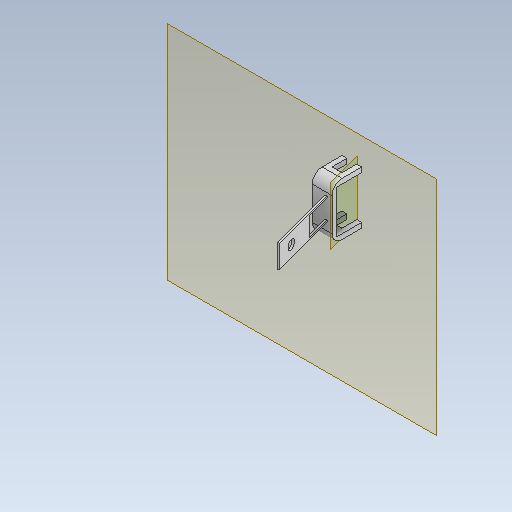
# Autodesk Inventor part: Кранштейн сервомоторов
Saved by Autodesk Inventor 2021.2 (Build 252289000, 289)
## iProperties
Created: 2021-10-14
Part Number: Кранштейн сервомоторов
Material: Типовые
Document SubType Name: Modeling
Designer: Surflay
Density: 1 g/cm^3
Appearance: По умолчанию
Author: Surflay
Autodesk Inventor part; units mm, degrees
ref_plane "YZ Plane" through (0, 0, 0) normal (1, 0, 0) x (0, 1, 0)
ref_plane "XZ Plane" through (0, 0, 0) normal (0, 1, 0) x (-1, 0, 0)
ref_plane "XY Plane" through (0, 0, 0) normal (0, 0, 1) x (1, 0, 0)
ref_plane "РабПлоскость1" through (0, 0, 0) normal (0, 0, 1) x (1, 0, 0)
sketch "Эскиз1" plane through (0, 0, 0) normal (0, 0, 1) x (1, 0, 0)
  line L0 (63.5, 74.8221) -> (63.5, 48.8221) projected
  line L1 (60.5, 48.8221) -> (60.5, 74.8221) projected
  line L2 (123.5, 102) -> (-123.5, 102) projected
  line L3 (43.5, 11.5) -> (33.5, 11.5) projected
  line L4 (68.5, 11.5) -> (43.5, 11.5) projected
  line L5 (40.5, 31.5) -> (60.5, 31.5)
  line L6 (60.5, 31.5) -> (60.5, 85)
  line L7 (60.5, 85) -> (40.5, 85)
  line L8 (40.5, 85) -> (40.5, 31.5)
  point P0 (0, 0)
  dimension "d0" = 20
  dimension "d1" = 17
  dimension "d2" = 0
  dimension "d3" = 20
  constraints: 8 end point, 2 parallel, 1 horizontal, 1 perpendicular
  measures "d0" distance from line of L3.start L5
  measures "d1" distance between parallel lines of L2 L7
  measures "d2" distance between parallel lines of L1 L6
  measures "d3" distance between parallel lines of L8 L6
extrude "Выдавливание1" add sketch "Эскиз1" along normal blind 30
ref_plane "РабПлоскость2" through (60.5, 31.5, 30) normal (-0.9659258, 0, 0.258819) x (0, 1, 0)
sketch "Эскиз2" plane through (60.5, 31.5, 30) normal (-0.9659258, 0, 0.258819) x (0, 1, 0)
  line L0 (46.5, -71.3991) -> (65.5, -71.3991) projected
  ellipse E0 centre (65.5, -66.5694) end of major axis (70.5, -66.5694) minor radius 4.8296 (65.5, -71.3991) -> (70.5, -66.5694) ccw projected
  line L1 (70.5, -66.5694) -> (70.5, -56.9102) projected
  ellipse E1 centre (65.5, -56.9102) end of major axis (70.5, -56.9102) minor radius 4.8296 (70.5, -56.9102) -> (65.5, -52.0805) ccw projected
  line L2 (65.5, -52.0805) -> (54.0465, -52.0805) projected
  ellipse E2 centre (54.0465, -42.4213) end of major axis (64.0465, -42.4213) minor radius 9.6593 (44.7292, -45.9289) -> (54.0465, -52.0805) ccw projected
  ellipse E3 centre (30.5, -51.2856) end of major axis (45.7717, -51.2856) minor radius 14.7513 (44.7292, -45.9289) -> (30.5, -36.5343) ccw projected
  line L3 (30.5, -36.5343) -> (-7.5, -36.5343) projected
  line L4 (-7.5, -36.5343) -> (-7.5, -31.008) projected
  ellipse E4 centre (6.5042, -17.2158) end of major axis (26.5042, -17.2158) minor radius 19.3185 (-12.2897, -23.8231) -> (-7.5, -31.008) ccw projected
  line L5 (-12.2897, -23.8231) -> (-15.4018, -15.5639) projected
  ellipse E5 centre (-20.1003, -17.2158) end of major axis (-15.1003, -17.2158) minor radius 4.8296 (-15.4018, -15.5639) -> (-20.1003, -12.3861) ccw projected
  line L6 (-20.1003, -12.3861) -> (-40.9046, -12.3861) projected
  ellipse E6 centre (-40.9046, -17.2158) end of major axis (-45.9046, -17.2158) minor radius 4.8296 (-40.9046, -12.3861) -> (-45.8286, -16.3771) ccw projected
  line L7 (-45.8286, -16.3771) -> (-50.2368, -40.5253) projected
  line L8 (-50.2368, -40.5253) -> (-52.0642, -60.7008) projected
  ellipse E7 centre (-47.0832, -61.1217) end of major axis (-52.0832, -61.1217) minor radius 4.8296 (-52.0642, -60.7008) -> (-47.519, -65.933) ccw projected
  line L9 (-47.519, -65.933) -> (14.9298, -71.2104) projected
  ellipse E8 centre (14.0582, -80.8329) end of major axis (4.0582, -80.8329) minor radius 9.6593 (18.7926, -72.3248) -> (14.9298, -71.2104) ccw projected
  ellipse E9 centre (30.5, -51.2856) end of major axis (55.2283, -51.2856) minor radius 23.8857 (18.7926, -72.3248) -> (41.8928, -72.4853) ccw projected
  ellipse E10 centre (46.5, -81.0583) end of major axis (36.5, -81.0583) minor radius 9.6593 (46.5, -71.3991) -> (41.8928, -72.4853) ccw projected
  ellipse E11 centre (30.3221, -55.759) end of major axis (33.8221, -55.759) minor radius 3.3807 projected
  line L10 (0, 0) -> (53.5, 0) projected
  line L11 (41.8928, 0) -> (18.7926, 0)
  line L12 (18.7926, 0) -> (18.7926, -70)
  line L13 (18.7926, -70) -> (41.8928, -70)
  line L14 (41.8928, -70) -> (41.8928, 0)
  circle A0 centre (30.5, -51.2856) radius 4.5
  ellipse E12 centre (30.3619, -58.823) end of major axis (44.3161, -58.823) minor radius 13.4788 (17.3132, -63.5994) -> (17.3137, -63.6006) ccw projected
  ellipse E13 centre (20.8132, -63.6558) end of major axis (17.3132, -63.6558) minor radius 3.3807 (18.8684, -66.4666) -> (17.3137, -63.6006) ccw projected
  ellipse E14 centre (30.3619, -58.823) end of major axis (44.3161, -58.823) minor radius 13.4788 (18.8684, -66.4666) -> (41.8272, -66.506) ccw projected
  ellipse E15 centre (39.8691, -63.7038) end of major axis (36.3691, -63.7038) minor radius 3.3807 (43.3691, -63.7038) -> (41.8272, -66.506) ccw projected
  line L15 (43.3691, -63.7038) -> (43.3691, -65.0724) projected
  ellipse E16 centre (30.3619, -60.1915) end of major axis (16.4077, -60.1915) minor radius 13.4788 (42.4671, -66.8966) -> (43.3691, -65.0724) ccw projected
  ellipse E17 centre (30.3619, -60.1915) end of major axis (16.4077, -60.1915) minor radius 13.4788 (18.2308, -66.8526) -> (42.4671, -66.8966) ccw projected
  ellipse E18 centre (30.3619, -60.1915) end of major axis (16.4077, -60.1915) minor radius 13.4788 (17.3132, -64.968) -> (18.2308, -66.8526) ccw projected
  line L16 (17.3132, -64.968) -> (17.3132, -63.6558) projected
  line L17 (17.3132, -63.6558) -> (17.3132, -63.5994) projected
  line L18 (25.6422, -60.4178) -> (35.002, -60.4178) projected
  ellipse E19 centre (30.3221, -64.0447) end of major axis (36.3221, -64.0447) minor radius 5.7956 (25.6422, -60.4178) -> (35.002, -60.4178) ccw projected
  point P0 (-31.5, 44.6363)
  dimension "d7" = 70
  dimension "d28" = 9
  constraints: 8 end point, 2 parallel, 1 centre point, 1 coincident, 1 horizontal, 1 perpendicular, 1 point on line, 19 other
  measures "d7" distance between parallel lines of L13 L10
  measures "d28" diameter of A0
extrude "Выдавливание2" add sketch "Эскиз2" along normal blind 10 contours L14 E15 E14 L13 E13 L12 L3 E3 | E3 L3 L12 L10 L14 | L14 E17 L13 E14 E15 | L14 L13 E17 | E13 E14 L13 E17 L12 | E17 L13 L12 | E11 A0 | L18 E19 picked at (30.1856, -56.8739)
sketch "Эскиз3" plane through (50.8407, 31.5, 32.5882) normal (-0.9659258, 0, 0.258819) x (0.258819, 0, 0.9659258)
  line L0 (70, 41.8928) -> (0, 41.8928) projected
  line L1 (0, 18.7926) -> (70, 18.7926) projected
  line L2 (70, 18.7926) -> (70, 41.8928) projected
  line L3 (0, 18.7926) -> (0, 41.8928) projected
  line L4 (0, 39.8928) -> (50, 39.8928)
  line L5 (50, 39.8928) -> (50, 20.7926)
  line L6 (50, 20.7926) -> (0, 20.7926)
  line L7 (0, 20.7926) -> (0, 39.8928)
  line L8 (50, 20.7926) -> (68, 20.7926)
  line L9 (68, 20.7926) -> (68, 39.8928)
  line L10 (68, 39.8928) -> (50, 39.8928)
  line L11 (52, 39.8928) -> (52, 20.7926)
  point P0 (-44.6363, -31.5)
  dimension "d10" = 2
  dimension "d11" = 2
  dimension "d12" = 2
  dimension "d13" = 50
  dimension "d14" = 2
  constraints: 16 end point, 4 perpendicular, 3 point on line, 2 horizontal, 2 parallel
  measures "d10" distance between parallel lines of L2 L9
  measures "d11" distance between parallel lines of L1 L8
  measures "d12" distance between parallel lines of L0 L10
  measures "d13" distance between parallel lines of L3 L5
  measures "d14" distance between parallel lines of L5 L11
extrude "Выдавливание3" cut sketch "Эскиз3" against normal blind 4 contours L4 L5 L6 L3 | L10 L9 L8 L11
sketch "Эскиз4" plane through (60.5, 31.5, 30) normal (0.9659258, 0, -0.258819) x (-0.258819, 0, -0.9659258)
  line L0 (-50, 20.7926) -> (0, 20.7926) projected
  line L1 (-68, 20.7926) -> (-52, 20.7926) projected
  line L2 (-68, 39.8928) -> (-68, 20.7926) projected
  line L3 (-52, 39.8928) -> (-68, 39.8928) projected
  line L4 (0, 39.8928) -> (-50, 39.8928) projected
  line L5 (-50, 39.8928) -> (-50, 20.7926) projected
  line L6 (-52, 20.7926) -> (-52, 39.8928) projected
  line L7 (0, 20.7926) -> (0, 39.8928)
  line L8 (0, 18.7926) -> (0, 41.8928) projected
  point P0 (44.6363, -31.5)
  constraints: 2 end point, 1 collinear
extrude "Выдавливание4" cut sketch "Эскиз4" against normal blind 4
sketch "Эскиз5" plane through (78.6173, 73.3928, 97.6148) normal (0, 1, 0) x (0.9659258, 0, -0.258819)
  line L0 (-4, 20) -> (-4, 70) projected
  line L1 (-6, 70) -> (-6, 20) projected
  line L2 (-6, 2) -> (-6, 18) projected
  line L3 (-4, 18) -> (-4, 2) projected
  line L4 (-10, 20) -> (-6, 20) projected
  line L5 (-10, 18) -> (-6, 18) projected
  line L6 (0, 18) -> (-4, 18) projected
  line L7 (0, 20) -> (-4, 20) projected
  line L8 (0, 70) -> (-10, 70) projected
  line L9 (0, 0) -> (-10, 0) projected
  line L10 (-2, 70) -> (-8, 70)
  line L11 (-8, 70) -> (-8, 0)
  line L12 (-8, 0) -> (-2, 0)
  line L13 (-2, 0) -> (-2, 70)
  line L14 (0, 0) -> (0, 70) projected
  line L15 (-10, 0) -> (-10, 70) projected
  line L16 (-4, 2) -> (-6, 2)
  line L17 (0, 0) -> (-10, 0) projected
  line L18 (-6, 70) -> (-4, 70)
  line L19 (-4, 70) -> (-4, 20)
  line L20 (-2, 20) -> (-4, 20)
  line L21 (-6, 20) -> (-6, 70) projected
  line L22 (-6, 20) -> (-8, 20)
  line L23 (-6, 20) -> (-6, 70)
  line L24 (0, 70) -> (-10, 70) projected
  line L25 (-6, 18) -> (-6, 2) projected
  line L26 (-6, 20) -> (-6, 2)
  line L27 (-4, 2) -> (-4, 18) projected
  line L28 (-6, 2) -> (-4, 2)
  line L29 (-4, 2) -> (-4, 20.7345)
  point P0 (-50.6739, 114.6363)
  point P1 (-4, 20)
  point P2 (-4, 18)
  point P3 (-6, 18)
  dimension "d19" = 2
  dimension "d20" = 2
  constraints: 26 end point, 5 point on line, 3 collinear, 3 parallel, 3 perpendicular, 2 midpoint, 1 horizontal, 1 vertical
  measures "d19" distance between parallel lines of L3 L13
  measures "d20" distance between parallel lines of L11 L2
extrude "Выдавливание5" cut sketch "Эскиз5" against normal through all contours L0 L8 L13 L7 | L7 L13 L6 L29 | L13 L8 L14 L7 | L7 L14 L6 L13 | L6 L13 L9 L11 L5 L2 L16 L3 | L6 L14 L9 L13 | L1 L4 L11 L8 | L26 L5 L11 L4 | L11 L4 L15 L8 | L9 L15 L5 L11 | L11 L5 L15 L4
sketch "Эскиз6" plane through (54.7044, 31.5, 31.5529) normal (-0.9659258, 0, 0.258819) x (0.258819, 0, 0.9659258)
  line L0 (68, 41.8928) -> (68, 18.7926) projected
  line L1 (0, 41.8928) -> (68, 41.8928) projected
  line L2 (0, 18.7926) -> (0, 41.8928) projected
  line L3 (68, 18.7926) -> (0, 18.7926) projected
  line L4 (0, 0) -> (0, 53.5) projected
  line L5 (0, 39.8928) -> (25, 39.8928)
  line L6 (25, 39.8928) -> (25, 20.7926)
  line L7 (25, 20.7926) -> (0, 20.7926)
  line L8 (0, 20.7926) -> (0, 39.8928)
  point P0 (-44.6363, -31.5)
  point P1 (0, 20.7926)
  dimension "d23" = 25
  dimension "d24" = 2
  dimension "d25" = 2
  constraints: 8 end point, 2 parallel, 1 horizontal, 1 perpendicular, 1 point on line
  measures "d23" distance of L6.end L7.end
  measures "d24" distance between parallel lines of L3 L7
  measures "d25" distance between parallel lines of L1 L5
extrude "Выдавливание6" cut sketch "Эскиз6" against normal through all contours L5 L6 L7 L2
sketch "Эскиз7" plane through (40.5, 31.5, 0) normal (-1, 0, 0) x (0, 0, 1)
  line L0 (0, 0) -> (0, 53.5) projected
  line L1 (0, 48.5) -> (25, 48.5)
  line L2 (25, 48.5) -> (25, 5)
  line L3 (25, 5) -> (0, 5)
  line L4 (0, 5) -> (0, 48.5)
  line L5 (30, 53.5) -> (30, 0) projected
  line L6 (0, 53.5) -> (30, 53.5) projected
  line L7 (0, 0) -> (30, 0) projected
  point P0 (0, -31.5)
  point P1 (0, 5)
  dimension "d29" = 5
  dimension "d30" = 5
  dimension "d31" = 5
  constraints: 8 end point, 2 parallel, 1 horizontal, 1 perpendicular, 1 point on line
  measures "d29" distance between parallel lines of L5 L2
  measures "d30" distance between parallel lines of L6 L1
  measures "d31" distance between parallel lines of L7 L3
extrude "Выдавливание7" cut sketch "Эскиз7" against normal through all contours L0 L1 L2 L3
fillet "Сопряжение1" radius 10 2 edges at (50.5, 85, 30) (50.5, 31.5, 30)
sketch "Эскиз8" plane through (40.5, 85, 0) normal (0, 1, 0) x (1, 0, 0)
  line L0 (20, 0) -> (0, 0) projected
  line L1 (15, 0) -> (5, 0)
  line L2 (5, 0) -> (5, -15)
  line L3 (5, -15) -> (15, -15)
  line L4 (15, -15) -> (15, 0)
  line L5 (20, -20) -> (0, -20) projected
  line L6 (0, 0) -> (0, -20) projected
  line L7 (20, 0) -> (20, -20) projected
  point P0 (-40.5, 0)
  point P1 (5, 0)
  dimension "d35" = 5
  dimension "d36" = 5
  dimension "d37" = 5
  constraints: 8 end point, 2 parallel, 1 horizontal, 1 perpendicular, 1 point on line
  measures "d35" distance between parallel lines of L5 L3
  measures "d36" distance between parallel lines of L6 L2
  measures "d37" distance between parallel lines of L7 L4
extrude "Выдавливание8" cut sketch "Эскиз8" against normal through all contours L4 L3 L2 L0
